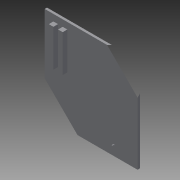
# Autodesk Inventor part: Base
Saved by Autodesk Inventor 2015 (Build 190159000, 159)
## iProperties
Created: 2015-04-16
Part Number: Base
Material: Generic
Document SubType Name: Modeling
Designer: WASHHSST
Density: 1 g/cm^3
Appearance: Default
Author: WASHHSST
Autodesk Inventor part; units mm, degrees
ref_plane "YZ Plane" through (0, 0, 0) normal (1, 0, 0) x (0, 1, 0)
ref_plane "XZ Plane" through (0, 0, 0) normal (0, 1, 0) x (-1, 0, 0)
ref_plane "XY Plane" through (0, 0, 0) normal (0, 0, 1) x (1, 0, 0)
sketch "Sketch1" plane through (0, 0, 0) normal (0, 0, 1) x (1, 0, 0)
  line L0 (0, 0) -> (508, 0)
  line L1 (508, 0) -> (508, 508)
  line L2 (508, 508) -> (0, 508)
  line L3 (0, 508) -> (0, 0)
  dimension "d0" = 508
  dimension "d1" = 508
  constraints: 8 end point, 2 parallel, 1 horizontal, 1 perpendicular
  measures "d0" distance of L2.end L1.end
  measures "d1" distance of L1.end L0.end
extrude "Extrusion1" add sketch "Sketch1" along normal blind 12.7
sketch "Sketch2" plane through (0, 0, 12.7) normal (0, 0, 1) x (1, 0, 0)
  circle A0 centre (51.0764, 55.0392) radius 3.175
  circle A1 centre (379.8659, 55.0392) radius 3.175
  point P0 (0, 0)
  dimension "d4" = 6.35
  dimension "d5" = 6.35
  constraints: 2 centre point
  measures "d4" diameter of A0
  measures "d5" diameter of A1
extrude "Extrusion2" add sketch "Sketch2" along normal blind 12.7
sketch "Sketch3" plane through (0, 0, 12.7) normal (0, 0, 1) x (1, 0, 0)
  line L0 (25.4, 495.3) -> (50.8, 495.3)
  line L1 (50.8, 495.3) -> (50.8, 292.1)
  line L2 (50.8, 292.1) -> (25.4, 292.1)
  line L3 (25.4, 292.1) -> (25.4, 495.3)
  line L4 (76.2, 495.3) -> (101.6, 495.3)
  line L5 (101.6, 495.3) -> (101.6, 292.1)
  line L6 (101.6, 292.1) -> (76.2, 292.1)
  line L7 (76.2, 292.1) -> (76.2, 495.3)
  line L8 (508, 508) -> (0, 508) projected
  line L9 (0, 508) -> (0, 0) projected
  dimension "d8" = 25.4
  dimension "d9" = 203.2
  dimension "d10" = 25.4
  dimension "d11" = 203.2
  dimension "d12" = 25.4
  dimension "d15" = 12.7
  dimension "d16" = 12.7
  dimension "d17" = 50.8
  constraints: 16 end point, 4 parallel, 2 horizontal, 2 perpendicular
  measures "d8" distance of L1.end L2.end
  measures "d9" distance of L0.end L1.end
  measures "d10" distance of L5.end L7.start
  measures "d11" distance of L4.end L5.end
  measures "d12" distance between parallel lines of L7 L1
  measures "d15" distance between parallel lines of L8 L0
  measures "d16" distance between parallel lines of L8 L4
  measures "d17" distance between parallel lines of L9 L1
extrude "Extrusion3" add sketch "Sketch3" along normal blind 25.4
body "Solid1"
